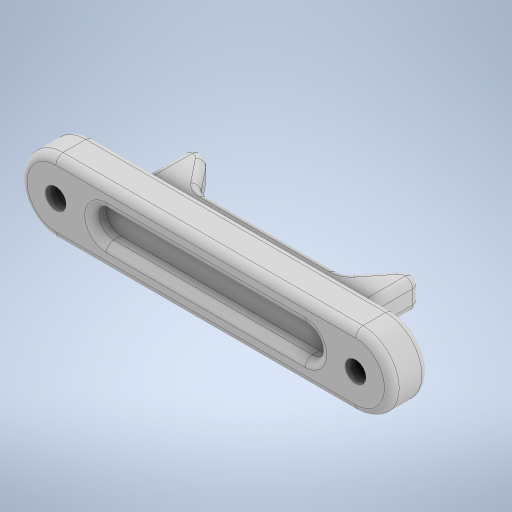
# Autodesk Inventor part: Front Shock Brace
Saved by Autodesk Inventor 2024 (Build 280153000, 153)
## iProperties
Created: 2023-07-03
Part Number: Front Shock Brace
Material: Generic
Document SubType Name: Modeling
Designer: patel
Density: 1 g/cm^3
Appearance: Default
Author: patel
Autodesk Inventor part; units mm, degrees
ref_plane "YZ Plane" through (0, 0, 0) normal (1, 0, 0) x (0, 1, 0)
ref_plane "XZ Plane" through (0, 0, 0) normal (0, 1, 0) x (-1, 0, 0)
sketch "Sketch1" plane through (0, 0, 0) normal (0, 0, 1) x (1, 0, 0)
  line L0 (-16.5735, 4.0005) -> (16.5735, 4.0005)
  line L1 (16.5735, 4.0005) -> (16.5735, -4.0005) construction
  line L2 (16.5735, -4.0005) -> (-16.5735, -4.0005)
  line L3 (-16.5735, -4.0005) -> (-16.5735, 4.0005) construction
  line L4 (-16.5735, 4.0005) -> (16.5735, -4.0005) construction
  line L5 (16.5735, 4.0005) -> (-16.5735, -4.0005) construction
  arc A0 (16.5735, -4.0005) -> (16.5735, 4.0005) centre (16.5735, 0) ccw
  arc A1 (-16.5735, 4.0005) -> (-16.5735, -4.0005) centre (-16.5735, 0) ccw
  point P0 (0, 0)
  dimension "d0" = 33.147
  dimension "d1" = 8.001
  dimension "d2" = 4.0005
  constraints: 12 end point, 4 point on circle, 2 centre point, 2 midpoint, 2 parallel, 1 equal radius, 1 horizontal, 1 perpendicular
  measures "d0" distance of L1.end L2.end
  measures "d1" distance of L0.end L1.end
  measures "d2" radius of A0
extrude "Extrusion1" add sketch "Sketch1" along normal blind 4.1275
sketch "Sketch2" plane through (0, 0, 4.1275) normal (0, 0, 1) x (1, 0, 0)
  line L0 (-10.9855, 1.5875) -> (10.9855, 1.5875)
  line L1 (10.9855, 1.5875) -> (10.9855, -1.5875) construction
  line L2 (10.9855, -1.5875) -> (-10.9855, -1.5875)
  line L3 (-10.9855, -1.5875) -> (-10.9855, 1.5875) construction
  line L4 (-10.9855, 1.5875) -> (10.9855, -1.5875) construction
  line L5 (10.9855, 1.5875) -> (-10.9855, -1.5875) construction
  arc A0 (-10.9855, 1.5875) -> (-10.9855, -1.5875) centre (-10.9855, 0) ccw
  arc A1 (10.9855, -1.5875) -> (10.9855, 1.5875) centre (10.9855, 0) ccw
  point P0 (0, 0)
  dimension "d5" = 21.971
  dimension "d6" = 3.175
  constraints: 12 end point, 4 point on circle, 4 tangent, 2 centre point, 2 midpoint, 2 parallel, 1 horizontal, 1 perpendicular
  measures "d5" distance of L1.end L2.end
  measures "d6" distance of L0.end L1.end
extrude "Extrusion2" cut sketch "Sketch2" against normal blind 1.5875
sketch "Sketch3" plane through (0, 0, 4.1275) normal (0, 0, 1) x (1, 0, 0)
  arc A0 (16.5735, -4.0005) -> (16.5735, 4.0005) centre (16.5735, 0) ccw projected
  arc A1 (-16.5735, 4.0005) -> (-16.5735, -4.0005) centre (-16.5735, 0) ccw projected
  point P0 (0, 0)
  constraints: 2 coincident
hole "Hole1" at (16.5735, 0, 4.1275) at (-16.5735, 0, 4.1275) direction (0, 0, -1) diameter 2.2708 end through all thread size "4-48 UNF" class "2B" standard "ANSI Unified Screw Threads"
ref_plane "Work Plane1" through (-16.5735, 0, -37.9939) normal (0, 1, 0) x (0, 0, 1)
sketch "Sketch5" plane through (-16.5735, 0, -37.9939) normal (0, 1, 0) x (0, 0, 1)
  line L0 (37.9939, 0) -> (37.9939, 33.147) projected
  line L1 (37.9939, 4.0005) -> (31.0089, 4.0005)
  line L2 (37.9939, 4.0005) -> (44.9789, 4.0005) construction
  line L3 (31.0089, 4.0005) -> (31.0089, 5.588)
  line L4 (31.0089, 5.588) -> (34.8189, 8.636)
  line L5 (34.8189, 8.636) -> (34.8189, 24.511)
  line L6 (37.9939, -4.0005) -> (42.1214, -4.0005) projected
  line L7 (28.2149, 16.5735) -> (47.7729, 16.5735) construction
  line L8 (37.9939, 29.1465) -> (31.0089, 29.1465)
  line L9 (31.0089, 29.1465) -> (31.0089, 27.559)
  line L10 (31.0089, 27.559) -> (34.8189, 24.511)
  line L11 (34.8189, 8.636) -> (34.8189, 24.511)
  point P0 (37.9939, 16.5735)
  point P1 (34.8189, 16.5735)
  point P2 (37.9939, 16.5735)
  dimension "d16" = 6.985
  dimension "d17" = 180
  dimension "d18" = 1.5875
  dimension "d19" = 15.875
  dimension "d20" = 3.175
  dimension "d21" = 8.001
  constraints: 18 end point, 3 symmetric about line, 2 collinear, 2 midpoint, 2 perpendicular, 1 horizontal, 1 horizontal alignment, 1 parallel, 1 point on line
  measures "d16" distance of L1.start L1.end
  measures "d17" angle of L1 L2
  measures "d18" distance of L1.end L3.end
  measures "d19" distance of L4.end L5.end
  measures "d20" distance between parallel lines of L0 L5
  measures "d21" distance between parallel lines of L6 L1
extrude "Extrusion3" add sketch "Sketch5" along normal mid plane 3.175
fillet "Fillet1" radius 1.5875 4 edges at (-7.9375, 0, -3.175) (-10.9855, 0, -6.985) (7.9375, 0, -3.175) (10.9855, 0, -6.985)
fillet "Fillet2" radius 0.8128 40 edges at (-12.573, 1.5875, -3.4925) (-11.0608, 1.5875, -6.8283) (-12.1607, 1.5875, -6.985) (-7.8622, 1.5875, -3.3317) (0, 1.5875, -3.175) (7.8622, 1.5875, -3.3317) (9.4615, 1.5875, -5.08) (11.0608, 1.5875, -6.8283) (12.1607, 1.5875, -6.985) (-9.4615, 1.5875, -5.08) (0, 1.5875, 0) (12.573, 1.5875, -3.4925) (12.573, 0, 0) (12.573, -1.5875, -3.4925) (12.573, 0, -6.985) (-12.573, 0, -6.985) (-12.573, 0, 0) (-12.573, -1.5875, -3.4925) (0, -1.5875, 0) (7.8622, -1.5875, -3.3317) (9.4615, -1.5875, -5.08) (11.0608, -1.5875, -6.8283) (12.1607, -1.5875, -6.985) (-7.8622, -1.5875, -3.3317) (-9.4615, -1.5875, -5.08) (-11.0608, -1.5875, -6.8283) (-12.1607, -1.5875, -6.985) (0, -1.5875, -3.175) (-20.574, 0, 0) (0, -4.0005, 0) (20.574, 0, 0) (0, 4.0005, 0) (-20.574, 0, 4.1275) (0, -4.0005, 4.1275) (20.574, 0, 4.1275) (0, 4.0005, 4.1275) (12.573, 0, 4.1275) (0, -1.5875, 4.1275) (-12.573, 0, 4.1275) (0, 1.5875, 4.1275)
body "Solid1"
